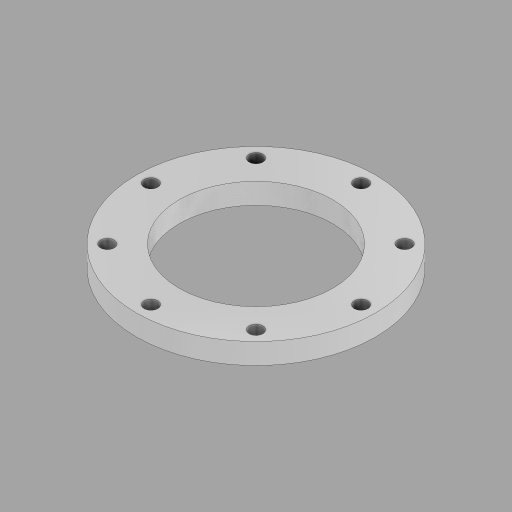
# Autodesk Inventor part: CollarRingBottom
Saved by Autodesk Inventor 2024 (Build 280153020, 153B)
## iProperties
Created: 2023-10-25
Part Number: CollarRingBottom
Material: Stainless Steel
Document SubType Name: Modeling
Designer: schanen
Density: 8 g/cm^3
Appearance: Polished - Small Pyramid Knurl
Author: schanen
Autodesk Inventor part; units mm, degrees
ref_plane "YZ Plane" through (0, 0, 0) normal (1, 0, 0) x (0, 1, 0)
ref_plane "XZ Plane" through (0, 0, 0) normal (0, 1, 0) x (-1, 0, 0)
ref_plane "XY Plane" through (0, 0, 0) normal (0, 0, 1) x (1, 0, 0)
sketch "Sketch1" plane through (0, 0, 0) normal (0, 0, 1) x (1, 0, 0)
  line L0 (-66.5, 0) -> (-103.5, 0)
  line L1 (-103.5, 0) -> (-103.5, 18)
  line L2 (-103.5, 18) -> (-66.5, 18)
  line L3 (-66.5, 18) -> (-66.5, 0)
  line L4 (0, -3.6) -> (0, 21.6) projected
  point P0 (0, 0)
  dimension "d0" = 66.5
  dimension "d1" = 103.5
  dimension "d2" = 18
  constraints: 8 end point, 2 parallel, 1 horizontal, 1 horizontal alignment, 1 perpendicular
  measures "d0" distance from line of point (0, 0) L3
  measures "d1" distance from line of point (0, 0) L1
  measures "d2" distance of L0.end L1.end
revolve "Revolution1" add sketch "Sketch1" angle 360 about axis through (0, -10, 0) along (0, 1, 0)
sketch "Sketch2" plane through (0, 18, 0) normal (0, 1, 0) x (1, 0, 0)
  point P0 (0, 0)
  point P1 (0, 91)
  dimension "d4" = 91
  measures "d4" distance of point (0, 0) point (0, 91)
hole "Hole1" at (0, 18, -91) direction (0, -1, 0) diameter 12 end through all
pattern_circular "Circular Pattern1" count 8 over 360 about axis through (0, 9, 0) along (0, 1, 0) of "Hole1"
body "Solid1"
